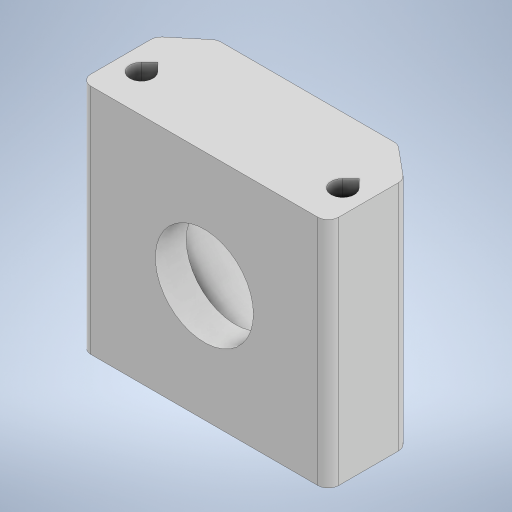
# Autodesk Inventor part: Uchwyt_na_lozysko_poli
Saved by Autodesk Inventor 2023 (Build 270158000, 158)
## iProperties
Created: 2023-01-27
Part Number: Uchwyt_na_lozysko_poli
Material: Generic
Document SubType Name: Modeling
Designer: Kamil
Density: 1 g/cm^3
Appearance: Default
Mass: 10.8368 g
Surface Area: 48.2707 cm^2
Volume: 10.8368 cm^3
Author: Kamil
Autodesk Inventor part; units mm, degrees
ref_plane "YZ Plane" through (0, 0, 0) normal (1, 0, 0) x (0, 1, 0)
ref_plane "XZ Plane" through (0, 0, 0) normal (0, 1, 0) x (-1, 0, 0)
ref_plane "XY Plane" through (0, 0, 0) normal (0, 0, 1) x (1, 0, 0)
sketch "Sketch1" plane through (0, 0, 0) normal (0, 0, 1) x (1, 0, 0)
  circle A0 centre (15, 0) radius 15 projected
  line L0 (15, 0) -> (15, 15)
  line L1 (15, 0) -> (15, 22.5)
  circle A1 centre (15, 0) radius 15
  circle A2 centre (15, 0) radius 22.5
  line L2 (30, 0) -> (39, 0)
  line L3 (0, 0) -> (-9, 0)
  line L4 (15, 0) -> (39, 0)
  line L5 (39, 0) -> (39, 22.5)
  line L6 (39, 22.5) -> (15, 22.5)
  line L7 (15, 22.5) -> (15, 0)
  line L8 (39, 22.5) -> (-9, 22.5)
  line L9 (-9, 22.5) -> (-9, 0)
  line L10 (-9, 0) -> (39, 0)
  line L11 (39, 0) -> (39, 22.5)
  circle A3 centre (15, 0) radius 12 projected
  dimension "d0" = 22.5
  dimension "d3" = 9
  dimension "d4" = 9
  constraints: 24 end point, 4 horizontal, 4 parallel, 3 point on circle, 2 coincident, 2 perpendicular, 1 centre point, 1 vertical, 1 vertical alignment, 2 other
  measures "d0" distance of L0.start L1.end
  measures "d3" distance of L2.start L2.end
  measures "d4" distance of L3.start L3.end
ref_plane "Work Plane1" through (-4.4951, -19.4951, -9) normal (0, 0, -1) x (0, 1, 0)
extrude "Extrusion1" add sketch "Sketch1" against normal up to surface (9 mm away) contours A0 L1 A2 L2 | A0 L3 A2 L1 | A2 L6 L5 L2 | A2 L3 L9 L8
sketch "Sketch2" plane through (0, 0, 0) normal (0, 0, 1) x (1, 0, 0)
  line L0 (39, 0) -> (39, 22.5) projected
  line L1 (39, 22.5) -> (-9, 22.5) projected
  line L2 (-9, 22.5) -> (-9, 0) projected
  line L3 (-9, 0) -> (0, 0) projected
  arc A0 (30, 0) -> (0, 0) centre (15, 0) ccw projected
  line L4 (30, 0) -> (39, 0) projected
  circle A1 centre (15, 0) radius 14.4 projected
  line L5 (3.2369, -3.5618) -> (3.2813, -3.7192) projected
  line L6 (3.2813, -3.7192) -> (1.8309, -4.1298) projected
  line L7 (1.8309, -4.1298) -> (1.6039, -3.3274) projected
  line L8 (1.6039, -3.3274) -> (1.7752, -3.279) projected
  line L9 (1.7752, -3.279) -> (1.9579, -3.924) projected
  line L10 (1.9579, -3.924) -> (2.4068, -3.7968) projected
  line L11 (2.4068, -3.7968) -> (2.2489, -3.2388) projected
  line L12 (2.2489, -3.2388) -> (2.4199, -3.1904) projected
  line L13 (2.4199, -3.1904) -> (2.5779, -3.7484) projected
  line L14 (2.5779, -3.7484) -> (3.2369, -3.5618) projected
  line L15 (2.1376, -0.6913) -> (2.1686, -1.0539) projected
  line L16 (2.1686, -1.0539) -> (1.9921, -1.0691) projected
  line L17 (1.9921, -1.0691) -> (1.9458, -0.5462) projected
  line L18 (1.9458, -0.5462) -> (2.5047, -0.4984) projected
  spline S0 degree 3 poles (2.5047, -0.4984) (2.5251, -0.5167) (2.5649, -0.5525) (2.618, -0.6104) (2.6642, -0.6698) (2.7032, -0.7309) (2.7348, -0.7936) (2.7589, -0.8578) (2.7762, -0.9236) (2.7815, -0.9684) (2.7841, -0.9909) knots 0 0 0 0 0.141618 0.276217 0.405435 0.529564 0.649766 0.767321 0.883595 1 1 1 1 projected
  spline S1 degree 3 poles (2.7841, -0.9909) (2.7851, -1.0058) (2.7872, -1.0353) (2.7863, -1.0791) (2.7831, -1.1219) (2.7767, -1.1638) (2.7672, -1.2048) (2.7552, -1.2449) (2.7396, -1.2837) (2.7219, -1.3217) (2.7008, -1.3582) (2.6771, -1.3933) (2.6504, -1.4266) (2.6211, -1.4583) (2.5891, -1.4885) (2.5542, -1.5168) (2.5167, -1.5436) (2.4766, -1.569) (2.4337, -1.592) (2.3884, -1.6128) (2.3408, -1.6314) (2.2905, -1.6471) (2.238, -1.6608) (2.183, -1.672) (2.1257, -1.6809) (2.0866, -1.6847) (2.0667, -1.6867) knots 0 0 0 0 0.039887 0.078907 0.116955 0.154508 0.192037 0.229148 0.266128 0.303579 0.341084 0.378733 0.416519 0.454867 0.493967 0.533828 0.574805 0.617052 0.660451 0.70458 0.750216 0.79683 0.845263 0.895052 0.946592 1 1 1 1 projected
  spline S2 degree 3 poles (2.0667, -1.6867) (2.0464, -1.6882) (2.0066, -1.6913) (1.9475, -1.6918) (1.8902, -1.6907) (1.8347, -1.6859) (1.7809, -1.6791) (1.729, -1.6689) (1.6787, -1.6562) (1.6304, -1.6407) (1.5845, -1.6228) (1.5409, -1.6035) (1.5007, -1.5816) (1.4629, -1.5585) (1.4283, -1.5329) (1.3963, -1.5059) (1.3672, -1.4769) (1.3413, -1.4459) (1.3176, -1.4133) (1.297, -1.3786) (1.279, -1.3421) (1.2635, -1.304) (1.2502, -1.2642) (1.24, -1.2226) (1.2323, -1.1792) (1.2293, -1.1496) (1.2278, -1.1345) knots 0 0 0 0 0.053942 0.105892 0.156508 0.205926 0.253698 0.300306 0.34613 0.391071 0.434954 0.476875 0.517214 0.556499 0.594234 0.63128 0.667439 0.702968 0.738447 0.774173 0.809921 0.846256 0.883109 0.9211 0.959905 1 1 1 1 projected
  spline S3 degree 3 poles (1.2278, -1.1345) (1.2263, -1.1125) (1.2235, -1.0697) (1.2282, -1.007) (1.2385, -0.9479) (1.2563, -0.8928) (1.2804, -0.8417) (1.3094, -0.7941) (1.3451, -0.7513) (1.3787, -0.7185) (1.4091, -0.6948) (1.434, -0.6773) (1.4616, -0.6614) (1.4911, -0.6458) (1.523, -0.6312) (1.5569, -0.6172) (1.5933, -0.6044) (1.6185, -0.5967) (1.6314, -0.5927) knots 0 0 0 0 0.088878 0.172965 0.252831 0.330221 0.405649 0.48026 0.554402 0.62994 0.668991 0.709858 0.7526 0.797447 0.844321 0.893869 0.945511 1 1 1 1 projected
  line L19 (1.6314, -0.5927) -> (1.6932, -0.7358) projected
  spline S4 degree 3 poles (1.6932, -0.7358) (1.6736, -0.7425) (1.6368, -0.7552) (1.5863, -0.777) (1.5442, -0.8006) (1.5092, -0.8256) (1.4807, -0.8535) (1.4562, -0.8838) (1.4361, -0.9179) (1.4192, -0.9546) (1.4068, -0.9941) (1.3992, -1.0358) (1.3961, -1.0793) (1.3977, -1.1089) (1.3985, -1.1239) knots 0 0 0 0 0.115925 0.217694 0.307764 0.385841 0.457769 0.530534 0.603423 0.678945 0.756397 0.834408 0.915859 1 1 1 1 projected
  spline S5 degree 3 poles (1.3985, -1.1239) (1.3997, -1.135) (1.402, -1.1567) (1.4079, -1.1884) (1.4154, -1.2188) (1.4253, -1.2477) (1.4367, -1.2755) (1.4506, -1.3017) (1.466, -1.3268) (1.4835, -1.3504) (1.503, -1.3727) (1.5248, -1.3934) (1.5485, -1.413) (1.5746, -1.4308) (1.6027, -1.4478) (1.6332, -1.4627) (1.6655, -1.477) (1.7002, -1.4892) (1.7367, -1.5003) (1.775, -1.5091) (1.8152, -1.5157) (1.857, -1.5206) (1.9006, -1.5232) (1.9459, -1.5242) (1.993, -1.523) (2.0249, -1.5205) (2.0411, -1.5193) knots 0 0 0 0 0.039283 0.077116 0.113656 0.149529 0.184819 0.219553 0.25411 0.288393 0.323135 0.358316 0.394422 0.431449 0.469807 0.509816 0.551167 0.594521 0.639354 0.685623 0.733159 0.782873 0.834148 0.887122 0.942608 1 1 1 1 projected
  spline S6 degree 3 poles (2.0411, -1.5193) (2.0655, -1.5168) (2.1127, -1.5122) (2.1807, -1.5001) (2.2438, -1.4851) (2.3018, -1.4663) (2.3546, -1.4438) (2.4026, -1.4179) (2.4455, -1.3884) (2.483, -1.3551) (2.5152, -1.3189) (2.5434, -1.2812) (2.5659, -1.241) (2.5836, -1.199) (2.597, -1.1552) (2.6047, -1.1091) (2.608, -1.0612) (2.6061, -1.0287) (2.6051, -1.0122) knots 0 0 0 0 0.08583 0.166283 0.241617 0.312644 0.379514 0.442649 0.503178 0.561584 0.617954 0.672615 0.726085 0.778955 0.832023 0.886125 0.942033 1 1 1 1 projected
  spline S7 degree 3 poles (2.6051, -1.0122) (2.603, -0.996) (2.5988, -0.9632) (2.5857, -0.9145) (2.5666, -0.866) (2.5425, -0.8183) (2.5148, -0.7731) (2.4845, -0.7326) (2.4532, -0.6966) (2.4296, -0.6769) (2.4182, -0.6673) knots 0 0 0 0 0.121865 0.246498 0.375835 0.510728 0.645128 0.770782 0.888853 1 1 1 1 projected
  line L20 (2.4182, -0.6673) -> (2.1376, -0.6913) projected
  line L21 (2.6025, 1.3397) -> (2.6783, 1.9399) projected
  line L22 (2.6783, 1.9399) -> (2.8542, 1.9177) projected
  line L23 (2.8542, 1.9177) -> (2.752, 1.1086) projected
  spline S8 degree 3 poles (2.752, 1.1086) (2.7429, 1.1097) (2.7246, 1.1118) (2.6969, 1.1182) (2.6688, 1.1267) (2.6401, 1.1374) (2.6109, 1.1502) (2.5815, 1.1659) (2.5514, 1.1836) (2.5203, 1.2033) (2.4889, 1.2269) (2.4562, 1.2534) (2.4225, 1.2838) (2.3879, 1.318) (2.3521, 1.3558) (2.3159, 1.3976) (2.2779, 1.4427) (2.2529, 1.4745) (2.24, 1.4909) knots 0 0 0 0 0.041688 0.084485 0.12957 0.176132 0.224349 0.275221 0.328483 0.384238 0.443657 0.507674 0.577026 0.651212 0.730351 0.814894 0.904522 1 1 1 1 projected
  spline S9 degree 3 poles (2.24, 1.4909) (2.2251, 1.51) (2.1966, 1.5465) (2.1546, 1.5985) (2.1145, 1.6453) (2.0775, 1.6877) (2.0422, 1.7246) (2.0098, 1.7569) (1.9798, 1.7845) (1.9434, 1.8136) (1.8998, 1.8432) (1.8479, 1.8709) (1.7968, 1.8908) (1.7621, 1.8968) (1.7454, 1.8997) knots 0 0 0 0 0.110149 0.211547 0.305173 0.391124 0.468427 0.538175 0.600133 0.654157 0.750871 0.839947 0.92244 1 1 1 1 projected
  spline S10 degree 3 poles (1.7454, 1.8997) (1.736, 1.9007) (1.7178, 1.9025) (1.6908, 1.9029) (1.665, 1.9007) (1.6401, 1.8965) (1.6162, 1.8901) (1.5934, 1.8812) (1.5715, 1.8703) (1.5514, 1.8567) (1.5321, 1.8422) (1.5155, 1.8254) (1.5002, 1.8082) (1.4879, 1.789) (1.4771, 1.769) (1.4685, 1.7476) (1.4625, 1.7248) (1.4599, 1.7092) (1.4586, 1.7013) knots 0 0 0 0 0.07208 0.140771 0.207341 0.271501 0.334551 0.397314 0.459449 0.522013 0.584309 0.644471 0.70314 0.761158 0.819468 0.878314 0.938146 1 1 1 1 projected
  spline S11 degree 3 poles (1.4586, 1.7013) (1.4577, 1.6927) (1.456, 1.6758) (1.4566, 1.6506) (1.4601, 1.6265) (1.4654, 1.6031) (1.4738, 1.5807) (1.4847, 1.5591) (1.4984, 1.5386) (1.5141, 1.5188) (1.5324, 1.5004) (1.5536, 1.4841) (1.5768, 1.4694) (1.6023, 1.4565) (1.6303, 1.4457) (1.6606, 1.4365) (1.6933, 1.4292) (1.716, 1.4259) (1.7277, 1.4243) knots 0 0 0 0 0.059655 0.117027 0.172817 0.227446 0.281886 0.337566 0.393632 0.451854 0.511205 0.57249 0.635363 0.700427 0.769528 0.841883 0.918584 1 1 1 1 projected
  line L24 (1.7277, 1.4243) -> (1.6891, 1.2721) projected
  spline S12 degree 3 poles (1.6891, 1.2721) (1.6718, 1.2758) (1.6384, 1.2829) (1.5908, 1.2979) (1.5466, 1.3144) (1.506, 1.3333) (1.4692, 1.3549) (1.436, 1.3787) (1.4066, 1.405) (1.381, 1.4337) (1.3589, 1.4643) (1.3406, 1.4968) (1.3255, 1.5309) (1.3146, 1.5668) (1.3072, 1.6042) (1.3037, 1.6432) (1.3036, 1.684) (1.3065, 1.7115) (1.308, 1.7256) knots 0 0 0 0 0.079519 0.15435 0.22545 0.292312 0.356633 0.417711 0.476803 0.5346 0.591095 0.646938 0.702987 0.75911 0.816116 0.875058 0.936035 1 1 1 1 projected
  spline S13 degree 3 poles (1.308, 1.7256) (1.3102, 1.7407) (1.3146, 1.7701) (1.3259, 1.8122) (1.3409, 1.8508) (1.3591, 1.8863) (1.3817, 1.918) (1.4072, 1.947) (1.4368, 1.9721) (1.4697, 1.9934) (1.5044, 2.0118) (1.5402, 2.0271) (1.5766, 2.0394) (1.6138, 2.0484) (1.6516, 2.0547) (1.6902, 2.0572) (1.7295, 2.0572) (1.7558, 2.0543) (1.7691, 2.0528) knots 0 0 0 0 0.0719 0.140341 0.205101 0.267236 0.328103 0.388491 0.44897 0.510883 0.573241 0.63419 0.694328 0.754511 0.814678 0.875189 0.936985 1 1 1 1 projected
  spline S14 degree 3 poles (1.7691, 2.0528) (1.7809, 2.0511) (1.8044, 2.0475) (1.8391, 2.0395) (1.8732, 2.0295) (1.9065, 2.0166) (1.9392, 2.0016) (1.9713, 1.9846) (2.0027, 1.965) (2.0339, 1.9428) (2.0658, 1.917) (2.0992, 1.8869) (2.135, 1.8527) (2.173, 1.8137) (2.2128, 1.77) (2.2552, 1.7217) (2.3, 1.6692) (2.3299, 1.6321) (2.3453, 1.613) knots 0 0 0 0 0.048063 0.095872 0.143222 0.191366 0.239486 0.288143 0.337726 0.388442 0.44253 0.502768 0.569571 0.642146 0.72202 0.808066 0.900891 1 1 1 1 projected
  spline S15 degree 3 poles (2.3453, 1.613) (2.355, 1.6009) (2.3735, 1.5778) (2.3997, 1.5446) (2.4242, 1.5152) (2.4458, 1.4888) (2.4652, 1.4657) (2.4825, 1.4461) (2.4972, 1.4297) (2.5205, 1.4052) (2.5541, 1.3737) (2.5867, 1.3508) (2.6025, 1.3397) knots 0 0 0 0 0.122963 0.235585 0.33712 0.427177 0.507413 0.577226 0.634969 0.682948 0.846402 1 1 1 1 projected
  spline S16 degree 3 poles (3.2126, 3.3885) (3.2081, 3.3748) (3.1992, 3.3477) (3.1797, 3.3099) (3.1556, 3.2755) (3.1266, 3.2449) (3.0933, 3.2175) (3.0552, 3.1937) (3.0125, 3.1735) (2.965, 3.1564) (2.9117, 3.1442) (2.8521, 3.1378) (2.786, 3.1369) (2.7135, 3.1413) (2.6345, 3.1517) (2.549, 3.1674) (2.4569, 3.1885) (2.3938, 3.2059) (2.361, 3.215) knots 0 0 0 0 0.044757 0.088212 0.13131 0.174466 0.218471 0.264535 0.313339 0.364759 0.420593 0.482299 0.550231 0.625199 0.707298 0.797101 0.894511 1 1 1 1 projected
  spline S17 degree 3 poles (2.361, 3.215) (2.3316, 3.2238) (2.2746, 3.2408) (2.193, 3.2696) (2.1175, 3.2992) (2.0487, 3.3309) (1.9861, 3.3636) (1.9299, 3.3979) (1.8803, 3.434) (1.8367, 3.4712) (1.8001, 3.5103) (1.7697, 3.5504) (1.7464, 3.592) (1.7295, 3.6349) (1.7196, 3.679) (1.7172, 3.7245) (1.7205, 3.7711) (1.7282, 3.8017) (1.7321, 3.8174) knots 0 0 0 0 0.094891 0.184012 0.267398 0.345466 0.418176 0.485934 0.548826 0.607777 0.662835 0.714172 0.76306 0.809854 0.856144 0.902359 0.950205 1 1 1 1 projected
  spline S18 degree 3 poles (1.7321, 3.8174) (1.7365, 3.8311) (1.7452, 3.8581) (1.7641, 3.8954) (1.7867, 3.9293) (1.8138, 3.9593) (1.8448, 3.9857) (1.88, 4.0083) (1.919, 4.0278) (1.9474, 4.037) (1.9619, 4.0417) knots 0 0 0 0 0.128572 0.252071 0.372106 0.49136 0.611467 0.734523 0.863694 1 1 1 1 projected
  spline S19 degree 3 poles (1.9619, 4.0417) (1.981, 4.0467) (2.0207, 4.0572) (2.0845, 4.0644) (2.1538, 4.0664) (2.2289, 4.0624) (2.3098, 4.0532) (2.3964, 4.0381) (2.4889, 4.0173) (2.552, 3.9997) (2.5847, 3.9906) knots 0 0 0 0 0.093485 0.19435 0.303629 0.42214 0.550467 0.689616 0.83904 1 1 1 1 projected
  spline S20 degree 3 poles (2.5847, 3.9906) (2.614, 3.9819) (2.6709, 3.9651) (2.7521, 3.9363) (2.8272, 3.9067) (2.8958, 3.8753) (2.9583, 3.8427) (3.0143, 3.8081) (3.0642, 3.7723) (3.1076, 3.735) (3.1444, 3.6961) (3.1751, 3.6562) (3.1984, 3.6145) (3.2152, 3.5717) (3.225, 3.5274) (3.2281, 3.4818) (3.2241, 3.4351) (3.2165, 3.4043) (3.2126, 3.3885) knots 0 0 0 0 0.094573 0.183468 0.266628 0.34434 0.417107 0.484651 0.547846 0.606844 0.661715 0.713282 0.762209 0.809039 0.855365 0.90195 0.949859 1 1 1 1 projected
  spline S21 degree 3 poles (2.9847, 2.4634) (2.9814, 2.4493) (2.9747, 2.4216) (2.958, 2.3826) (2.9367, 2.3464) (2.9107, 2.3132) (2.8793, 2.2837) (2.8432, 2.2569) (2.8023, 2.2334) (2.7564, 2.2126) (2.7044, 2.196) (2.6455, 2.1852) (2.5798, 2.1789) (2.5071, 2.178) (2.4275, 2.1822) (2.3411, 2.1912) (2.2476, 2.2049) (2.1832, 2.2175) (2.1498, 2.2241) knots 0 0 0 0 0.04464 0.088342 0.13107 0.174304 0.218582 0.264447 0.31322 0.364612 0.420422 0.481931 0.549885 0.625078 0.706968 0.796771 0.894376 1 1 1 1 projected
  spline S22 degree 3 poles (2.1498, 2.2241) (2.1198, 2.2306) (2.0617, 2.2432) (1.9779, 2.265) (1.9005, 2.2889) (1.8294, 2.3151) (1.7645, 2.343) (1.7057, 2.3727) (1.6535, 2.4047) (1.6071, 2.4384) (1.5674, 2.4743) (1.534, 2.5119) (1.5076, 2.5516) (1.4873, 2.5929) (1.4747, 2.6364) (1.4676, 2.6813) (1.4681, 2.7282) (1.4732, 2.7594) (1.4759, 2.7753) knots 0 0 0 0 0.094852 0.184048 0.267512 0.345443 0.418244 0.485883 0.548846 0.60765 0.662738 0.714099 0.762746 0.809759 0.855923 0.902251 0.949945 1 1 1 1 projected
  spline S23 degree 3 poles (1.4759, 2.7753) (1.4792, 2.7894) (1.4856, 2.8168) (1.5016, 2.8555) (1.5212, 2.8911) (1.546, 2.923) (1.5747, 2.9519) (1.6082, 2.977) (1.6457, 2.9991) (1.6731, 3.0106) (1.6872, 3.0164) knots 0 0 0 0 0.128448 0.251708 0.372284 0.491264 0.611809 0.734772 0.864012 1 1 1 1 projected
  spline S24 degree 3 poles (1.6872, 3.0164) (1.7058, 3.0228) (1.7446, 3.0361) (1.8075, 3.0488) (1.8765, 3.0561) (1.9517, 3.0585) (2.0331, 3.055) (2.1208, 3.0471) (2.2146, 3.0336) (2.2788, 3.0211) (2.3121, 3.0146) knots 0 0 0 0 0.093434 0.194221 0.303629 0.42206 0.550623 0.689764 0.83947 1 1 1 1 projected
  spline S25 degree 3 poles (2.3121, 3.0146) (2.3419, 3.0081) (2.3998, 2.9956) (2.4831, 2.9737) (2.5602, 2.9496) (2.6313, 2.924) (2.6959, 2.8959) (2.7547, 2.8663) (2.8072, 2.8344) (2.8534, 2.8006) (2.8933, 2.765) (2.9266, 2.7274) (2.9531, 2.6878) (2.9733, 2.6463) (2.9865, 2.6029) (2.9929, 2.5577) (2.9926, 2.5108) (2.9874, 2.4794) (2.9847, 2.4634) knots 0 0 0 0 0.094629 0.183297 0.266536 0.344427 0.417005 0.484703 0.54799 0.606846 0.661773 0.713178 0.761869 0.808924 0.855219 0.901853 0.94959 1 1 1 1 projected
  spline S26 degree 3 poles (1.212, 0.6828) (1.2128, 0.6943) (1.2144, 0.7169) (1.2206, 0.75) (1.2298, 0.7814) (1.2415, 0.8114) (1.2566, 0.8397) (1.2747, 0.8662) (1.2955, 0.8913) (1.3193, 0.9147) (1.3458, 0.936) (1.3749, 0.9551) (1.4067, 0.9714) (1.4411, 0.9856) (1.4781, 0.9969) (1.5176, 1.0062) (1.5598, 1.0124) (1.5888, 1.0149) (1.6038, 1.0161) knots 0 0 0 0 0.060587 0.119249 0.176546 0.232878 0.288549 0.344691 0.401586 0.460123 0.519762 0.580349 0.642935 0.707601 0.775847 0.846582 0.921134 1 1 1 1 projected
  line L25 (1.6038, 1.0161) -> (1.6108, 0.8646) projected
  spline S27 degree 3 poles (1.6108, 0.8646) (1.5925, 0.8618) (1.5586, 0.8566) (1.5122, 0.844) (1.4734, 0.8293) (1.4522, 0.8153) (1.4424, 0.8089) knots 0 0 0 0 0.30893 0.575011 0.804592 1 1 1 1 projected
  spline S28 degree 3 poles (1.4424, 0.8089) (1.4364, 0.8041) (1.4246, 0.7949) (1.4096, 0.7787) (1.3959, 0.7624) (1.3849, 0.7449) (1.3764, 0.7264) (1.3696, 0.7073) (1.3652, 0.6872) (1.3642, 0.6734) (1.3636, 0.6664) knots 0 0 0 0 0.136071 0.266454 0.39235 0.514197 0.633868 0.754476 0.87465 1 1 1 1 projected
  spline S29 degree 3 poles (1.3636, 0.6664) (1.3635, 0.6555) (1.3633, 0.634) (1.3702, 0.6026) (1.3815, 0.5725) (1.3986, 0.544) (1.4209, 0.517) (1.4482, 0.4913) (1.481, 0.4673) (1.5053, 0.4533) (1.5179, 0.446) knots 0 0 0 0 0.114401 0.2257 0.336654 0.452128 0.573646 0.70444 0.846587 1 1 1 1 projected
  spline S30 degree 3 poles (1.5179, 0.446) (1.5301, 0.4398) (1.5554, 0.4269) (1.5969, 0.4116) (1.6422, 0.3969) (1.6923, 0.3855) (1.7465, 0.375) (1.805, 0.367) (1.8679, 0.3605) (1.9113, 0.3579) (1.9337, 0.3565) knots 0 0 0 0 0.095624 0.198388 0.309369 0.429113 0.557839 0.695566 0.842654 1 1 1 1 projected
  spline S31 degree 3 poles (1.9337, 0.3565) (1.9185, 0.3662) (1.8889, 0.3851) (1.8495, 0.4182) (1.8165, 0.4547) (1.7901, 0.4941) (1.7694, 0.5353) (1.7554, 0.5778) (1.7473, 0.6211) (1.7474, 0.6502) (1.7474, 0.6649) knots 0 0 0 0 0.14307 0.277636 0.406221 0.531242 0.652339 0.769982 0.884252 1 1 1 1 projected
  spline S32 degree 3 poles (1.7474, 0.6649) (1.7484, 0.6769) (1.7502, 0.7007) (1.7583, 0.7356) (1.7706, 0.7691) (1.7868, 0.8012) (1.8072, 0.8319) (1.8316, 0.8611) (1.8602, 0.889) (1.8926, 0.9152) (1.9282, 0.9392) (1.967, 0.9598) (2.0084, 0.9767) (2.0524, 0.9902) (2.0991, 0.9998) (2.1483, 1.0062) (2.2003, 1.009) (2.2358, 1.0079) (2.2539, 1.0073) knots 0 0 0 0 0.053131 0.105509 0.15752 0.210207 0.26388 0.319858 0.378143 0.439919 0.50353 0.567456 0.63334 0.700789 0.770371 0.843546 0.919805 1 1 1 1 projected
  spline S33 degree 3 poles (2.2539, 1.0073) (2.2786, 1.0055) (2.3268, 1.0019) (2.3969, 0.9879) (2.4631, 0.9676) (2.515, 0.9449) (2.5539, 0.924) (2.581, 0.9077) (2.606, 0.8903) (2.6289, 0.8721) (2.6497, 0.8527) (2.6686, 0.8327) (2.6855, 0.8117) (2.7047, 0.7827) (2.7244, 0.7449) (2.7402, 0.697) (2.7496, 0.6474) (2.7493, 0.6137) (2.7492, 0.5967) knots 0 0 0 0 0.103272 0.202419 0.298495 0.393049 0.438856 0.483081 0.525506 0.56631 0.605691 0.644161 0.681647 0.718409 0.789661 0.859117 0.929033 1 1 1 1 projected
  spline S34 degree 3 poles (2.7492, 0.5967) (2.7479, 0.5814) (2.7454, 0.5514) (2.7356, 0.5078) (2.7202, 0.4666) (2.6995, 0.4277) (2.6742, 0.3908) (2.6431, 0.3568) (2.6071, 0.3248) (2.5659, 0.2952) (2.5185, 0.2687) (2.4643, 0.2466) (2.4032, 0.2289) (2.3355, 0.215) (2.261, 0.2054) (2.1796, 0.2003) (2.0915, 0.1987) (2.0305, 0.2008) (1.9989, 0.2019) knots 0 0 0 0 0.048358 0.095019 0.140868 0.186898 0.233671 0.282017 0.332198 0.385487 0.44203 0.503407 0.569944 0.642621 0.721508 0.807294 0.899951 1 1 1 1 projected
  spline S35 degree 3 poles (1.9989, 0.2019) (1.9637, 0.204) (1.8961, 0.2079) (1.7989, 0.2181) (1.7097, 0.2321) (1.6284, 0.2491) (1.555, 0.2699) (1.4898, 0.2946) (1.4324, 0.3224) (1.383, 0.354) (1.3406, 0.3883) (1.3044, 0.4247) (1.274, 0.4629) (1.2492, 0.5031) (1.2309, 0.5455) (1.2184, 0.5897) (1.2113, 0.6357) (1.2118, 0.667) (1.212, 0.6828) knots 0 0 0 0 0.102611 0.19754 0.285012 0.3658 0.439695 0.507127 0.568796 0.625353 0.677945 0.727535 0.774719 0.82014 0.864669 0.908973 0.953834 1 1 1 1 projected
  line L26 (3.0025, -2.6804) -> (3.0347, -2.8508) projected
  line L27 (3.0347, -2.8508) -> (1.4687, -2.6642) projected
  line L28 (1.4687, -2.6642) -> (1.4361, -2.492) projected
  line L29 (1.4361, -2.492) -> (2.8204, -1.7164) projected
  line L30 (2.8204, -1.7164) -> (2.8551, -1.8999) projected
  line L31 (2.8551, -1.8999) -> (2.4339, -2.1258) projected
  line L32 (2.4339, -2.1258) -> (2.5298, -2.632) projected
  line L33 (2.5298, -2.632) -> (3.0025, -2.6804) projected
  circle A2 centre (15, 0) radius 12 projected
  arc A3 (30, 0) -> (0, 0) centre (15, 0) ccw projected
  line L34 (30, 0) -> (0, 0)
  circle A4 centre (15, 0) radius 10.4878
  point P0 (4.5122, 0)
  point P1 (25.4878, 0)
  point P2 (0, 0)
  constraints: 2 end point, 1 centre point, 1 coincident, 1 horizontal, 1 point on circle
extrude "Extrusion2" add sketch "Sketch2" along normal blind 2.8 contours L4 A0 L3 L2 L1 L0 | L34 A1 A0 | L34 A2 A1 | L34 A4 A2 picked at (8.2989, 11.7303) picked at (3.6203, 0.9573)
sketch "Sketch3" plane through (0, 0, 2.8) normal (0, 0, 1) x (1, 0, 0)
  line L0 (25.4878, 0) -> (39, 0) projected
  line L1 (39, 0) -> (39, 22.5) projected
  line L2 (39, 22.5) -> (-9, 22.5) projected
  line L3 (-9, 22.5) -> (-9, 0) projected
  line L4 (-9, 0) -> (4.5122, 0) projected
  arc A0 (25.4878, 0) -> (4.5122, 0) centre (15, 0) ccw projected
  spline S0 degree 3 poles (1.212, 0.6828) (1.2128, 0.6943) (1.2144, 0.7169) (1.2206, 0.75) (1.2298, 0.7814) (1.2415, 0.8114) (1.2566, 0.8397) (1.2747, 0.8662) (1.2955, 0.8913) (1.3193, 0.9147) (1.3458, 0.936) (1.3749, 0.9551) (1.4067, 0.9714) (1.4411, 0.9856) (1.4781, 0.9969) (1.5176, 1.0062) (1.5598, 1.0124) (1.5888, 1.0149) (1.6038, 1.0161) knots 0 0 0 0 0.060587 0.119249 0.176546 0.232878 0.288549 0.344691 0.401586 0.460123 0.519762 0.580349 0.642935 0.707601 0.775847 0.846582 0.921134 1 1 1 1 projected
  line L5 (1.6038, 1.0161) -> (1.6108, 0.8646) projected
  spline S1 degree 3 poles (1.6108, 0.8646) (1.5925, 0.8618) (1.5586, 0.8566) (1.5122, 0.844) (1.4734, 0.8293) (1.4522, 0.8153) (1.4424, 0.8089) knots 0 0 0 0 0.30893 0.575011 0.804592 1 1 1 1 projected
  spline S2 degree 3 poles (1.4424, 0.8089) (1.4364, 0.8041) (1.4246, 0.7949) (1.4096, 0.7787) (1.3959, 0.7624) (1.3849, 0.7449) (1.3764, 0.7264) (1.3696, 0.7073) (1.3652, 0.6872) (1.3642, 0.6734) (1.3636, 0.6664) knots 0 0 0 0 0.136071 0.266454 0.39235 0.514197 0.633868 0.754476 0.87465 1 1 1 1 projected
  spline S3 degree 3 poles (1.3636, 0.6664) (1.3635, 0.6555) (1.3633, 0.634) (1.3702, 0.6026) (1.3815, 0.5725) (1.3986, 0.544) (1.4209, 0.517) (1.4482, 0.4913) (1.481, 0.4673) (1.5053, 0.4533) (1.5179, 0.446) knots 0 0 0 0 0.114401 0.2257 0.336654 0.452128 0.573646 0.70444 0.846587 1 1 1 1 projected
  spline S4 degree 3 poles (1.5179, 0.446) (1.5301, 0.4398) (1.5554, 0.4269) (1.5969, 0.4116) (1.6422, 0.3969) (1.6923, 0.3855) (1.7465, 0.375) (1.805, 0.367) (1.8679, 0.3605) (1.9113, 0.3579) (1.9337, 0.3565) knots 0 0 0 0 0.095624 0.198388 0.309369 0.429113 0.557839 0.695566 0.842654 1 1 1 1 projected
  spline S5 degree 3 poles (1.9337, 0.3565) (1.9185, 0.3662) (1.8889, 0.3851) (1.8495, 0.4182) (1.8165, 0.4547) (1.7901, 0.4941) (1.7694, 0.5353) (1.7554, 0.5778) (1.7473, 0.6211) (1.7474, 0.6502) (1.7474, 0.6649) knots 0 0 0 0 0.14307 0.277636 0.406221 0.531242 0.652339 0.769982 0.884252 1 1 1 1 projected
  spline S6 degree 3 poles (1.7474, 0.6649) (1.7484, 0.6769) (1.7502, 0.7007) (1.7583, 0.7356) (1.7706, 0.7691) (1.7868, 0.8012) (1.8072, 0.8319) (1.8316, 0.8611) (1.8602, 0.889) (1.8926, 0.9152) (1.9282, 0.9392) (1.967, 0.9598) (2.0084, 0.9767) (2.0524, 0.9902) (2.0991, 0.9998) (2.1483, 1.0062) (2.2003, 1.009) (2.2358, 1.0079) (2.2539, 1.0073) knots 0 0 0 0 0.053131 0.105509 0.15752 0.210207 0.26388 0.319858 0.378143 0.439919 0.50353 0.567456 0.63334 0.700789 0.770371 0.843546 0.919805 1 1 1 1 projected
  spline S7 degree 3 poles (2.2539, 1.0073) (2.2786, 1.0055) (2.3268, 1.0019) (2.3969, 0.9879) (2.4631, 0.9676) (2.515, 0.9449) (2.5539, 0.924) (2.581, 0.9077) (2.606, 0.8903) (2.6289, 0.8721) (2.6497, 0.8527) (2.6686, 0.8327) (2.6855, 0.8117) (2.7047, 0.7827) (2.7244, 0.7449) (2.7402, 0.697) (2.7496, 0.6474) (2.7493, 0.6137) (2.7492, 0.5967) knots 0 0 0 0 0.103272 0.202419 0.298495 0.393049 0.438856 0.483081 0.525506 0.56631 0.605691 0.644161 0.681647 0.718409 0.789661 0.859117 0.929033 1 1 1 1 projected
  spline S8 degree 3 poles (2.7492, 0.5967) (2.7479, 0.5814) (2.7454, 0.5514) (2.7356, 0.5078) (2.7202, 0.4666) (2.6995, 0.4277) (2.6742, 0.3908) (2.6431, 0.3568) (2.6071, 0.3248) (2.5659, 0.2952) (2.5185, 0.2687) (2.4643, 0.2466) (2.4032, 0.2289) (2.3355, 0.215) (2.261, 0.2054) (2.1796, 0.2003) (2.0915, 0.1987) (2.0305, 0.2008) (1.9989, 0.2019) knots 0 0 0 0 0.048358 0.095019 0.140868 0.186898 0.233671 0.282017 0.332198 0.385487 0.44203 0.503407 0.569944 0.642621 0.721508 0.807294 0.899951 1 1 1 1 projected
  spline S9 degree 3 poles (1.9989, 0.2019) (1.9637, 0.204) (1.8961, 0.2079) (1.7989, 0.2181) (1.7097, 0.2321) (1.6284, 0.2491) (1.555, 0.2699) (1.4898, 0.2946) (1.4324, 0.3224) (1.383, 0.354) (1.3406, 0.3883) (1.3044, 0.4247) (1.274, 0.4629) (1.2492, 0.5031) (1.2309, 0.5455) (1.2184, 0.5897) (1.2113, 0.6357) (1.2118, 0.667) (1.212, 0.6828) knots 0 0 0 0 0.102611 0.19754 0.285012 0.3658 0.439695 0.507127 0.568796 0.625353 0.677945 0.727535 0.774719 0.82014 0.864669 0.908973 0.953834 1 1 1 1 projected
  spline S10 degree 3 poles (2.9847, 2.4634) (2.9814, 2.4493) (2.9747, 2.4216) (2.958, 2.3826) (2.9367, 2.3464) (2.9107, 2.3132) (2.8793, 2.2837) (2.8432, 2.2569) (2.8023, 2.2334) (2.7564, 2.2126) (2.7044, 2.196) (2.6455, 2.1852) (2.5798, 2.1789) (2.5071, 2.178) (2.4275, 2.1822) (2.3411, 2.1912) (2.2476, 2.2049) (2.1832, 2.2175) (2.1498, 2.2241) knots 0 0 0 0 0.04464 0.088342 0.13107 0.174304 0.218582 0.264447 0.31322 0.364612 0.420422 0.481931 0.549885 0.625078 0.706968 0.796771 0.894376 1 1 1 1 projected
  spline S11 degree 3 poles (2.1498, 2.2241) (2.1198, 2.2306) (2.0617, 2.2432) (1.9779, 2.265) (1.9005, 2.2889) (1.8294, 2.3151) (1.7645, 2.343) (1.7057, 2.3727) (1.6535, 2.4047) (1.6071, 2.4384) (1.5674, 2.4743) (1.534, 2.5119) (1.5076, 2.5516) (1.4873, 2.5929) (1.4747, 2.6364) (1.4676, 2.6813) (1.4681, 2.7282) (1.4732, 2.7594) (1.4759, 2.7753) knots 0 0 0 0 0.094852 0.184048 0.267512 0.345443 0.418244 0.485883 0.548846 0.60765 0.662738 0.714099 0.762746 0.809759 0.855923 0.902251 0.949945 1 1 1 1 projected
  spline S12 degree 3 poles (1.4759, 2.7753) (1.4792, 2.7894) (1.4856, 2.8168) (1.5016, 2.8555) (1.5212, 2.8911) (1.546, 2.923) (1.5747, 2.9519) (1.6082, 2.977) (1.6457, 2.9991) (1.6731, 3.0106) (1.6872, 3.0164) knots 0 0 0 0 0.128448 0.251708 0.372284 0.491264 0.611809 0.734772 0.864012 1 1 1 1 projected
  spline S13 degree 3 poles (1.6872, 3.0164) (1.7058, 3.0228) (1.7446, 3.0361) (1.8075, 3.0488) (1.8765, 3.0561) (1.9517, 3.0585) (2.0331, 3.055) (2.1208, 3.0471) (2.2146, 3.0336) (2.2788, 3.0211) (2.3121, 3.0146) knots 0 0 0 0 0.093434 0.194221 0.303629 0.42206 0.550623 0.689764 0.83947 1 1 1 1 projected
  spline S14 degree 3 poles (2.3121, 3.0146) (2.3419, 3.0081) (2.3998, 2.9956) (2.4831, 2.9737) (2.5602, 2.9496) (2.6313, 2.924) (2.6959, 2.8959) (2.7547, 2.8663) (2.8072, 2.8344) (2.8534, 2.8006) (2.8933, 2.765) (2.9266, 2.7274) (2.9531, 2.6878) (2.9733, 2.6463) (2.9865, 2.6029) (2.9929, 2.5577) (2.9926, 2.5108) (2.9874, 2.4794) (2.9847, 2.4634) knots 0 0 0 0 0.094629 0.183297 0.266536 0.344427 0.417005 0.484703 0.54799 0.606846 0.661773 0.713178 0.761869 0.808924 0.855219 0.901853 0.94959 1 1 1 1 projected
  spline S15 degree 3 poles (3.2126, 3.3885) (3.2081, 3.3748) (3.1992, 3.3477) (3.1797, 3.3099) (3.1556, 3.2755) (3.1266, 3.2449) (3.0933, 3.2175) (3.0552, 3.1937) (3.0125, 3.1735) (2.965, 3.1564) (2.9117, 3.1442) (2.8521, 3.1378) (2.786, 3.1369) (2.7135, 3.1413) (2.6345, 3.1517) (2.549, 3.1674) (2.4569, 3.1885) (2.3938, 3.2059) (2.361, 3.215) knots 0 0 0 0 0.044757 0.088212 0.13131 0.174466 0.218471 0.264535 0.313339 0.364759 0.420593 0.482299 0.550231 0.625199 0.707298 0.797101 0.894511 1 1 1 1 projected
  spline S16 degree 3 poles (2.361, 3.215) (2.3316, 3.2238) (2.2746, 3.2408) (2.193, 3.2696) (2.1175, 3.2992) (2.0487, 3.3309) (1.9861, 3.3636) (1.9299, 3.3979) (1.8803, 3.434) (1.8367, 3.4712) (1.8001, 3.5103) (1.7697, 3.5504) (1.7464, 3.592) (1.7295, 3.6349) (1.7196, 3.679) (1.7172, 3.7245) (1.7205, 3.7711) (1.7282, 3.8017) (1.7321, 3.8174) knots 0 0 0 0 0.094891 0.184012 0.267398 0.345466 0.418176 0.485934 0.548826 0.607777 0.662835 0.714172 0.76306 0.809854 0.856144 0.902359 0.950205 1 1 1 1 projected
  spline S17 degree 3 poles (1.7321, 3.8174) (1.7365, 3.8311) (1.7452, 3.8581) (1.7641, 3.8954) (1.7867, 3.9293) (1.8138, 3.9593) (1.8448, 3.9857) (1.88, 4.0083) (1.919, 4.0278) (1.9474, 4.037) (1.9619, 4.0417) knots 0 0 0 0 0.128572 0.252071 0.372106 0.49136 0.611467 0.734523 0.863694 1 1 1 1 projected
  spline S18 degree 3 poles (1.9619, 4.0417) (1.981, 4.0467) (2.0207, 4.0572) (2.0845, 4.0644) (2.1538, 4.0664) (2.2289, 4.0624) (2.3098, 4.0532) (2.3964, 4.0381) (2.4889, 4.0173) (2.552, 3.9997) (2.5847, 3.9906) knots 0 0 0 0 0.093485 0.19435 0.303629 0.42214 0.550467 0.689616 0.83904 1 1 1 1 projected
  spline S19 degree 3 poles (2.5847, 3.9906) (2.614, 3.9819) (2.6709, 3.9651) (2.7521, 3.9363) (2.8272, 3.9067) (2.8958, 3.8753) (2.9583, 3.8427) (3.0143, 3.8081) (3.0642, 3.7723) (3.1076, 3.735) (3.1444, 3.6961) (3.1751, 3.6562) (3.1984, 3.6145) (3.2152, 3.5717) (3.225, 3.5274) (3.2281, 3.4818) (3.2241, 3.4351) (3.2165, 3.4043) (3.2126, 3.3885) knots 0 0 0 0 0.094573 0.183468 0.266628 0.34434 0.417107 0.484651 0.547846 0.606844 0.661715 0.713282 0.762209 0.809039 0.855365 0.90195 0.949859 1 1 1 1 projected
  line L6 (2.6025, 1.3397) -> (2.6783, 1.9399) projected
  line L7 (2.6783, 1.9399) -> (2.8542, 1.9177) projected
  line L8 (2.8542, 1.9177) -> (2.752, 1.1086) projected
  spline S20 degree 3 poles (2.752, 1.1086) (2.7429, 1.1097) (2.7246, 1.1118) (2.6969, 1.1182) (2.6688, 1.1267) (2.6401, 1.1374) (2.6109, 1.1502) (2.5815, 1.1659) (2.5514, 1.1836) (2.5203, 1.2033) (2.4889, 1.2269) (2.4562, 1.2534) (2.4225, 1.2838) (2.3879, 1.318) (2.3521, 1.3558) (2.3159, 1.3976) (2.2779, 1.4427) (2.2529, 1.4745) (2.24, 1.4909) knots 0 0 0 0 0.041688 0.084485 0.12957 0.176132 0.224349 0.275221 0.328483 0.384238 0.443657 0.507674 0.577026 0.651212 0.730351 0.814894 0.904522 1 1 1 1 projected
  spline S21 degree 3 poles (2.24, 1.4909) (2.2251, 1.51) (2.1966, 1.5465) (2.1546, 1.5985) (2.1145, 1.6453) (2.0775, 1.6877) (2.0422, 1.7246) (2.0098, 1.7569) (1.9798, 1.7845) (1.9434, 1.8136) (1.8998, 1.8432) (1.8479, 1.8709) (1.7968, 1.8908) (1.7621, 1.8968) (1.7454, 1.8997) knots 0 0 0 0 0.110149 0.211547 0.305173 0.391124 0.468427 0.538175 0.600133 0.654157 0.750871 0.839947 0.92244 1 1 1 1 projected
  spline S22 degree 3 poles (1.7454, 1.8997) (1.736, 1.9007) (1.7178, 1.9025) (1.6908, 1.9029) (1.665, 1.9007) (1.6401, 1.8965) (1.6162, 1.8901) (1.5934, 1.8812) (1.5715, 1.8703) (1.5514, 1.8567) (1.5321, 1.8422) (1.5155, 1.8254) (1.5002, 1.8082) (1.4879, 1.789) (1.4771, 1.769) (1.4685, 1.7476) (1.4625, 1.7248) (1.4599, 1.7092) (1.4586, 1.7013) knots 0 0 0 0 0.07208 0.140771 0.207341 0.271501 0.334551 0.397314 0.459449 0.522013 0.584309 0.644471 0.70314 0.761158 0.819468 0.878314 0.938146 1 1 1 1 projected
  spline S23 degree 3 poles (1.4586, 1.7013) (1.4577, 1.6927) (1.456, 1.6758) (1.4566, 1.6506) (1.4601, 1.6265) (1.4654, 1.6031) (1.4738, 1.5807) (1.4847, 1.5591) (1.4984, 1.5386) (1.5141, 1.5188) (1.5324, 1.5004) (1.5536, 1.4841) (1.5768, 1.4694) (1.6023, 1.4565) (1.6303, 1.4457) (1.6606, 1.4365) (1.6933, 1.4292) (1.716, 1.4259) (1.7277, 1.4243) knots 0 0 0 0 0.059655 0.117027 0.172817 0.227446 0.281886 0.337566 0.393632 0.451854 0.511205 0.57249 0.635363 0.700427 0.769528 0.841883 0.918584 1 1 1 1 projected
  line L9 (1.7277, 1.4243) -> (1.6891, 1.2721) projected
  spline S24 degree 3 poles (1.6891, 1.2721) (1.6718, 1.2758) (1.6384, 1.2829) (1.5908, 1.2979) (1.5466, 1.3144) (1.506, 1.3333) (1.4692, 1.3549) (1.436, 1.3787) (1.4066, 1.405) (1.381, 1.4337) (1.3589, 1.4643) (1.3406, 1.4968) (1.3255, 1.5309) (1.3146, 1.5668) (1.3072, 1.6042) (1.3037, 1.6432) (1.3036, 1.684) (1.3065, 1.7115) (1.308, 1.7256) knots 0 0 0 0 0.079519 0.15435 0.22545 0.292312 0.356633 0.417711 0.476803 0.5346 0.591095 0.646938 0.702987 0.75911 0.816116 0.875058 0.936035 1 1 1 1 projected
  spline S25 degree 3 poles (1.308, 1.7256) (1.3102, 1.7407) (1.3146, 1.7701) (1.3259, 1.8122) (1.3409, 1.8508) (1.3591, 1.8863) (1.3817, 1.918) (1.4072, 1.947) (1.4368, 1.9721) (1.4697, 1.9934) (1.5044, 2.0118) (1.5402, 2.0271) (1.5766, 2.0394) (1.6138, 2.0484) (1.6516, 2.0547) (1.6902, 2.0572) (1.7295, 2.0572) (1.7558, 2.0543) (1.7691, 2.0528) knots 0 0 0 0 0.0719 0.140341 0.205101 0.267236 0.328103 0.388491 0.44897 0.510883 0.573241 0.63419 0.694328 0.754511 0.814678 0.875189 0.936985 1 1 1 1 projected
  spline S26 degree 3 poles (1.7691, 2.0528) (1.7809, 2.0511) (1.8044, 2.0475) (1.8391, 2.0395) (1.8732, 2.0295) (1.9065, 2.0166) (1.9392, 2.0016) (1.9713, 1.9846) (2.0027, 1.965) (2.0339, 1.9428) (2.0658, 1.917) (2.0992, 1.8869) (2.135, 1.8527) (2.173, 1.8137) (2.2128, 1.77) (2.2552, 1.7217) (2.3, 1.6692) (2.3299, 1.6321) (2.3453, 1.613) knots 0 0 0 0 0.048063 0.095872 0.143222 0.191366 0.239486 0.288143 0.337726 0.388442 0.44253 0.502768 0.569571 0.642146 0.72202 0.808066 0.900891 1 1 1 1 projected
  spline S27 degree 3 poles (2.3453, 1.613) (2.355, 1.6009) (2.3735, 1.5778) (2.3997, 1.5446) (2.4242, 1.5152) (2.4458, 1.4888) (2.4652, 1.4657) (2.4825, 1.4461) (2.4972, 1.4297) (2.5205, 1.4052) (2.5541, 1.3737) (2.5867, 1.3508) (2.6025, 1.3397) knots 0 0 0 0 0.122963 0.235585 0.33712 0.427177 0.507413 0.577226 0.634969 0.682948 0.846402 1 1 1 1 projected
  point P0 (0, 0)
  constraints: 28 other
extrude "Extrusion3" add sketch "Sketch3" against normal up to surface (2.8 mm away) contours S0 L5 S1 S2 S3 S4 S5 S6 S7 S8 S9 | S10 S11 S12 S13 S14 | S15 S16 S17 S18 S19 | L6 L7 L8 S20 S21 S22 S23 L9 S24 S25 S26 S27
sketch "Sketch4" plane through (39, 22.5, -9) normal (0, 0, -1) x (-1, 0, 0)
  line L0 (0, 0) -> (48, 0) projected
  line L1 (0, -22.5) -> (0, 0) projected
  line L2 (9, -22.5) -> (0, -22.5) projected
  arc A0 (39, -22.5) -> (9, -22.5) centre (24, -22.5) ccw projected
  line L3 (48, -22.5) -> (39, -22.5) projected
  line L4 (48, 0) -> (48, -22.5) projected
  line L5 (13.5122, -22.5) -> (0, -22.5) projected
  line L6 (0, -22.5) -> (0, 0) projected
  line L7 (0, 0) -> (48, 0) projected
  line L8 (48, 0) -> (48, -22.5) projected
  line L9 (48, -22.5) -> (34.4878, -22.5) projected
  arc A1 (34.4878, -22.5) -> (13.5122, -22.5) centre (24, -22.5) ccw projected
  point P0 (39, -22.5)
extrude "Extrusion4" add sketch "Sketch4" along normal blind 2.8
sketch "Sketch5" plane through (25.4878, 0, 0) normal (0, -1, 0) x (1, 0, 0)
  line L0 (13.5122, 2.8) -> (13.5122, -11.8) projected
  line L1 (0, 2.8) -> (13.5122, 2.8) projected
  line L2 (0, 0) -> (0, 2.8) projected
  line L3 (0, 0) -> (4.5122, 0) projected
  line L4 (4.5122, 0) -> (4.5122, -9) projected
  line L5 (4.5122, -9) -> (0, -9) projected
  line L6 (0, -9) -> (0, -11.8) projected
  line L7 (13.5122, -11.8) -> (0, -11.8) projected
  line L8 (-25.4878, 0) -> (-25.4878, -9) projected
  line L9 (-25.4878, 0) -> (-20.9756, 0) projected
  line L10 (-20.9756, 0) -> (-20.9756, 2.8) projected
  line L11 (-34.4878, 2.8) -> (-20.9756, 2.8) projected
  line L12 (-34.4878, -11.8) -> (-34.4878, 2.8) projected
  line L13 (-20.9756, -11.8) -> (-34.4878, -11.8) projected
  line L14 (-20.9756, -9) -> (-20.9756, -11.8) projected
  line L15 (-20.9756, -9) -> (-25.4878, -9) projected
  line L16 (0, -9) -> (-20.9756, -9) projected
  line L17 (-20.9756, -9) -> (-20.9756, -11.8) projected
  line L18 (0, -11.8) -> (-20.9756, -11.8) projected
  line L19 (0, -9) -> (0, -11.8) projected
  line L20 (0, -11.8) -> (-20.9756, -11.8) projected
  line L21 (-10.4878, -11.8) -> (-10.4878, 13.0665)
  line L22 (13.5122, 2.8) -> (13.5122, -11.8) projected
  line L23 (13.5122, -4.5) -> (4.5122, -4.5)
  line L24 (4.5122, 0) -> (4.5122, -9) projected
  circle A0 centre (9.0122, -4.5) radius 2
  circle A1 centre (9.0122, -4.5) radius 7.3
  line L25 (0, 2.8) -> (13.5122, 2.8) projected
  circle A2 centre (-29.9878, -4.5) radius 2
  circle A3 centre (-29.9878, -4.5) radius 7.3
  point P0 (-34.4878, 1.248)
  point P1 (-29.9878, 2.8)
  point P2 (-29.9878, -11.8)
  point P3 (-34.4878, -10.248)
  point P4 (13.5122, -10.248)
  point P5 (9.0122, -11.8)
  point P6 (9.0122, 2.8)
  point P7 (13.5122, 1.248)
  dimension "d13" = 4
  constraints: 4 centre point, 4 end point, 4 midpoint, 2 coincident, 2 symmetric about line, 1 tangent, 1 vertical, 2 other
  measures "d13" diameter of A0
extrude "Extrusion5" cut sketch "Sketch5" against normal through all contours L0 A1 L1 | L0 L7 A1 | A0 L23 | L23 A0 | L13 L12 A3 | L12 L11 A3 | A2
fillet "Fillet1" radius 2 4 edges at (39, 11.25, 1.248) (39, 11.25, -10.248) (-9, 11.25, -10.248) (-9, 11.25, 1.248)
mirror "Odbij1" about plane through (0, 0, 0) normal (0, -1, 0)
sketch "Szkic6" plane through (0, 0, 2.8) normal (0, 0, 1) x (1, 0, 0)
  circle A0 centre (15, 0) radius 15 projected
  circle A1 centre (15, 0) radius 10.4878 projected
  circle A2 centre (15, 0) radius 3.9811
  point P0 (0, 0)
  constraints: 1 centre point, 1 coincident
extrude "Wyciągnięcie proste6" add sketch "Szkic6" against normal up to surface (14.6 mm away) contours A0 | A1
sketch "Szkic7" plane through (-4.5, 22.5, 2.8) normal (0, 1, 0) x (1, 0, 0)
  circle A0 centre (39, 7.3) radius 2 projected
  circle A1 centre (0, 7.3) radius 2 projected
  arc A2 (-4.5, 2.6267) -> (-3.4434, 0.8632) centre (-2.5, 2.6267) ccw projected
  arc A3 (-3.4434, 0.8632) -> (0, 0) centre (0, 7.3) ccw projected
  line L0 (39, 0) -> (0, 0) projected
  arc A4 (39, 0) -> (42.4434, 0.8632) centre (39, 7.3) ccw projected
  arc A5 (42.4434, 0.8632) -> (43.5, 2.6267) centre (41.5, 2.6267) ccw projected
  line L1 (43.5, 2.6267) -> (43.5, 11.9733) projected
  arc A6 (43.5, 11.9733) -> (42.4434, 13.7368) centre (41.5, 11.9733) ccw projected
  arc A7 (42.4434, 13.7368) -> (39, 14.6) centre (39, 7.3) ccw projected
  line L2 (0, 14.6) -> (39, 14.6) projected
  arc A8 (0, 14.6) -> (-3.4434, 13.7368) centre (0, 7.3) ccw projected
  arc A9 (-3.4434, 13.7368) -> (-4.5, 11.9733) centre (-2.5, 11.9733) ccw projected
  line L3 (-4.5, 11.9733) -> (-4.5, 2.6267) projected
  line L4 (-4.5, 14.6) -> (43.5, 14.6)
  line L5 (43.5, 14.6) -> (43.5, 0)
  line L6 (43.5, 0) -> (-4.5, 0)
  line L7 (-4.5, 0) -> (-4.5, 14.6)
  point P0 (4.5, 2.8)
  point P1 (-4.5, 2.6267)
  point P2 (0, 0)
  point P3 (-4.5, 11.9733)
  point P4 (43.5, 2.6267)
  point P5 (39, 14.6)
  constraints: 8 end point, 2 parallel, 1 horizontal, 1 perpendicular, 1 point on line
extrude "Wyciągnięcie proste7" add sketch "Szkic7" against normal up to surface (45 mm away) contours A2 A3 L6 L7 | L7 L4 A8 A9 | A4 A5 L5 L6 | L4 L5 A6 A7
sketch "Szkic8" plane through (39, 22.5, -11.8) normal (0, 0, -1) x (-1, 0, 0)
  circle A0 centre (24, -22.5) radius 15
  point P0 (39, -22.5)
  constraints: 1 horizontal alignment, 2 other
extrude "Wyciągnięcie proste8" cut sketch "Szkic8" against normal blind 8.6
sketch "Szkic9" plane through (15, 0, -3.2) normal (0, 0, -1) x (-1, 0, 0)
  circle A0 centre (0, 0) radius 5
  circle A1 centre (0, 0) radius 12
  circle A2 centre (0, 0) radius 12
  circle A3 centre (0, 0) radius 7
  line L0 (0, 7) -> (0, 12)
  circle A4 centre (0, 0) radius 9.5
  point P0 (15, 0)
  constraints: 3 centre point, 2 end point, 2 vertical alignment, 1 coincident, 1 vertical, 10 other
extrude "Wyciągnięcie proste9" cut sketch "Szkic9" against normal through all contours A0 | A3 | A4
sketch "Szkic11" plane through (39, 22.5, -11.8) normal (0, 0, -1) x (-1, 0, 0)
  circle A0 centre (24, -22.5) radius 15 projected
  line L0 (0, 0) -> (48, 0) projected
  line L1 (48, -45) -> (0, -45) projected
  line L2 (48, 0) -> (48, -45) projected
  line L3 (0, 0) -> (0, -45) projected
  point P0 (39, -22.5)
ref_plane "Płaszczyzna konstrukcyjna2" through (1, -14, -17.2) normal (0, 0, -1) x (0, 1, 0)
extrude "Wyciągnięcie proste11" add sketch "Szkic11" along normal up to surface (5.4 mm away)
sketch "Szkic13" plane through (-9, -22.5, 2.8) normal (0, -1, 0) x (1, 0, 0)
  circle A0 centre (43.5, -7.3) radius 2 projected
  circle A1 centre (4.5, -7.3) radius 2 projected
  line L0 (0, 0) -> (0, -20) projected
  line L1 (0, -20) -> (48, -20) projected
  line L2 (48, 0) -> (48, -20) projected
  line L3 (48, 0) -> (0, 0) projected
  circle A2 centre (43.5, -7.3) radius 2 projected
  line L4 (0, 0) -> (43.5, 0)
  line L5 (0, -7.3) -> (0, 0)
  line L6 (43.5, -14.6) -> (0, -14.6)
  line L7 (0, -20) -> (0, 0) projected
  line L8 (48, 0) -> (48, -20) projected
  line L9 (43.5, 0) -> (48, 0)
  line L10 (48, 0) -> (48, -14.6)
  line L11 (48, -14.6) -> (43.5, -14.6)
  line L12 (9, -20) -> (39, -20) projected
  line L13 (9, -20) -> (39, -20) projected
  line L14 (39, -6) -> (9, -6) projected
  line L15 (9, -6) -> (9, -20)
  line L16 (9, -20) -> (39, -20)
  line L17 (39, -20) -> (39, -6)
  line L18 (39, -6) -> (9, -6) projected
  line L19 (24, -6) -> (24, -10)
  line L20 (39, -20) -> (41.5, -20)
  line L21 (48, -20) -> (0, -20) projected
  line L22 (9, -20) -> (6.5, -20)
  line L23 (0, -14.6) -> (6.5, -20)
  line L24 (48, -14.6) -> (41.5, -20)
  point P0 (9, -2.8)
  point P1 (0, -14.6)
  point P2 (48, -14.6)
  dimension "d40" = 2.5
  constraints: 28 end point, 3 point on line, 2 horizontal, 2 parallel, 2 perpendicular, 2 symmetric about line, 1 midpoint, 1 vertical
  measures "d40" distance of L16.end L20.end
extrude "Wyciągnięcie proste14" cut sketch "Szkic13" against normal through all contours L23 L1 L0 | L2 L1 L24
fillet "Zaokrąglenie7" radius 2 4 edges at (39, 0, -11.8) (32.5, 0, -17.2) (-2.5, 0, -17.2) (-9, 0, -11.8)
fillet "Zaokrąglenie8" radius 2 2 edges at (39, 0, 2.8) (-9, 0, 2.8)
sketch "Szkic15" plane through (31.7776, 22.5, -17.2) normal (0, 0, -1) x (-1, 0, 0)
  circle A0 centre (16.7776, -22.5) radius 15 projected
  line L0 (33.5552, 0) -> (33.5552, -45) projected
  line L1 (0, 0) -> (33.5552, 0) projected
  line L2 (0, -45) -> (0, 0) projected
  line L3 (33.5552, -45) -> (0, -45) projected
  circle A1 centre (16.7776, -22.5) radius 15.25
  point P0 (31.7776, -22.5)
  dimension "d50" = 30.5
  constraints: 1 centre point, 1 coincident
  measures "d50" diameter of A1
extrude "Wyciągnięcie proste16" cut sketch "Szkic15" against normal up to surface (14 mm away) contours A1
sketch "Szkic16" plane through (-1.7776, 22.5, -17.2) normal (0, 1, 0) x (1, 0, 0)
  line L0 (1.5276, -14) -> (32.0276, -14) projected
  circle A0 centre (-2.7224, -12.7) radius 2 projected
  circle A1 centre (36.2776, -12.7) radius 2 projected
  arc A2 (-7.2224, -18) -> (-5.2224, -20) centre (-5.2224, -18) ccw projected
  line L1 (-5.2224, -20) -> (38.7776, -20) projected
  arc A3 (38.7776, -20) -> (40.7776, -18) centre (38.7776, -18) ccw projected
  line L2 (40.7776, -18) -> (40.7776, -6.3386) projected
  arc A4 (40.7776, -6.3386) -> (40.0557, -4.8002) centre (38.7776, -6.3386) ccw projected
  line L3 (40.0557, -4.8002) -> (34.8333, -0.4616) projected
  arc A5 (34.8333, -0.4616) -> (33.5552, 0) centre (33.5552, -2) ccw projected
  line L4 (33.5552, 0) -> (0, 0) projected
  arc A6 (0, 0) -> (-1.278, -0.4616) centre (0, -2) ccw projected
  line L5 (-1.278, -0.4616) -> (-6.5004, -4.8002) projected
  arc A7 (-6.5004, -4.8002) -> (-7.2224, -6.3386) centre (-5.2224, -6.3386) ccw projected
  line L6 (-7.2224, -6.3386) -> (-7.2224, -18) projected
  circle A8 centre (-2.7224, -12.7) radius 2 projected
  circle A9 centre (-2.7224, -12.7) radius 2.25
  circle A10 centre (36.2776, -12.7) radius 2.25
  point P0 (1.7776, -17.2)
  dimension "d53" = 4.5
  dimension "d54" = 4.5
  constraints: 2 centre point, 2 coincident
  measures "d53" diameter of A9
  measures "d54" diameter of A10
extrude "Wyciągnięcie proste17" cut sketch "Szkic16" against normal through all contours A9 | A10
sketch "Szkic17" plane through (-1.7776, 22.5, -17.2) normal (0, 1, 0) x (1, 0, 0)
  circle A0 centre (36.2776, -12.7) radius 2.25 projected
  circle A1 centre (-2.7224, -12.7) radius 2.25 projected
  arc A2 (-7.2224, -18) -> (-5.2224, -20) centre (-5.2224, -18) ccw projected
  line L0 (-5.2224, -20) -> (38.7776, -20) projected
  arc A3 (38.7776, -20) -> (40.7776, -18) centre (38.7776, -18) ccw projected
  line L1 (40.7776, -18) -> (40.7776, -6.3386) projected
  arc A4 (40.7776, -6.3386) -> (40.0557, -4.8002) centre (38.7776, -6.3386) ccw projected
  line L2 (40.0557, -4.8002) -> (34.8333, -0.4616) projected
  arc A5 (34.8333, -0.4616) -> (33.5552, 0) centre (33.5552, -2) ccw projected
  line L3 (33.5552, 0) -> (0, 0) projected
  arc A6 (0, 0) -> (-1.278, -0.4616) centre (0, -2) ccw projected
  line L4 (-1.278, -0.4616) -> (-6.5004, -4.8002) projected
  arc A7 (-6.5004, -4.8002) -> (-7.2224, -6.3386) centre (-5.2224, -6.3386) ccw projected
  line L5 (-7.2224, -6.3386) -> (-7.2224, -18) projected
  line L6 (-2.7224, -12.7) -> (-2.7224, -8.4523)
  line L7 (-2.7224, -8.4523) -> (-6.0187, -13.7306)
  line L8 (-2.7224, -8.4523) -> (0.7467, -14.0073)
  circle A8 centre (-2.7224, -12.7) radius 2.25 projected
  line L9 (1.5276, 0) -> (32.0276, 0) projected
  line L10 (16.7776, 0) -> (16.7776, -20)
  line L11 (36.2776, -8.4523) -> (39.5739, -13.7306)
  line L12 (36.2776, -8.4523) -> (32.8085, -14.0073)
  point P0 (1.7776, -17.2)
  point P1 (34.3692, -11.5082)
  point P2 (38.186, -11.5082)
  point P3 (-4.6308, -11.5082)
  point P4 (-0.814, -11.5082)
  constraints: 12 end point, 3 symmetric about line, 2 midpoint, 2 tangent, 2 vertical
extrude "Wyciągnięcie proste18" cut sketch "Szkic17" against normal through all contours A0 L12 L11 | A1 L6 L8 | L7 L6 A1
sketch "Szkic18" plane through (-1.7776, 22.5, -17.2) normal (0, 1, 0) x (1, 0, 0)
  line L0 (36.2776, -8.4523) -> (38.186, -11.5082) projected
  arc A0 (34.3692, -11.5082) -> (38.186, -11.5082) centre (36.2776, -12.7) ccw projected
  line L1 (34.3692, -11.5082) -> (36.2776, -8.4523) projected
  line L2 (-2.7224, -8.4523) -> (-0.814, -11.5082) projected
  arc A1 (-4.6308, -11.5082) -> (-0.814, -11.5082) centre (-2.7224, -12.7) ccw projected
  line L3 (-4.6308, -11.5082) -> (-2.7224, -8.4523) projected
  arc A2 (-7.2224, -18) -> (-5.2224, -20) centre (-5.2224, -18) ccw projected
  line L4 (-5.2224, -20) -> (38.7776, -20) projected
  arc A3 (38.7776, -20) -> (40.7776, -18) centre (38.7776, -18) ccw projected
  line L5 (40.7776, -18) -> (40.7776, -6.3386) projected
  arc A4 (40.7776, -6.3386) -> (40.0557, -4.8002) centre (38.7776, -6.3386) ccw projected
  line L6 (40.0557, -4.8002) -> (34.8333, -0.4616) projected
  arc A5 (34.8333, -0.4616) -> (33.5552, 0) centre (33.5552, -2) ccw projected
  line L7 (33.5552, 0) -> (0, 0) projected
  arc A6 (0, 0) -> (-1.278, -0.4616) centre (0, -2) ccw projected
  line L8 (-1.278, -0.4616) -> (-6.5004, -4.8002) projected
  arc A7 (-6.5004, -4.8002) -> (-7.2224, -6.3386) centre (-5.2224, -6.3386) ccw projected
  line L9 (-7.2224, -6.3386) -> (-7.2224, -18) projected
  line L10 (-2.7224, -8.4523) -> (-2.7224, -12.7)
  line L11 (-5.7624, -12.558) -> (-2.7224, -9.518)
  line L12 (-2.7224, -9.518) -> (0.2108, -12.4512)
  line L13 (-2.7224, -9.518) -> (-2.7224, -19.476)
  circle A8 centre (-2.7224, -12.7) radius 2.25
  line L14 (16.7776, -20) -> (16.7776, -16.2297)
  line L15 (39.3176, -12.558) -> (36.2776, -9.518)
  line L16 (36.2776, -9.518) -> (33.3444, -12.4512)
  circle A9 centre (36.2776, -12.7) radius 2.25
  point P0 (1.7776, -17.2)
  point P1 (34.6866, -11.109)
  point P2 (37.8686, -11.109)
  point P3 (-4.3134, -11.109)
  point P4 (-1.1314, -11.109)
  dimension "d59" = 45
  dimension "d60" = 45
  constraints: 14 end point, 4 symmetric about line, 3 vertical, 2 centre point, 2 tangent, 1 coincident, 1 concentric, 1 midpoint, 1 other
  measures "d59" angle of L12 L13
  measures "d60" angle of L11 L13
extrude "Wyciągnięcie proste19" add sketch "Szkic18" against normal up to surface (45 mm away) contours L0 L15 L16 L1 | L0 A9 L15 | L16 A9 L1 | L10 L11 L3 | L2 L12 L10 | L2 A8 L12 | L11 A8 L3
body "Solid1"
